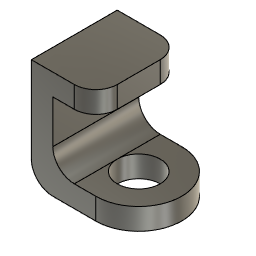
excercise 3 (Autodesk Fusion 360 design; units mm, degrees)
Autodesk Fusion 360 part; units mm, degrees
sketch "Sketch2" plane through (0, 0, 0) normal (0, 1, 0) x (1, 0, 0)
  line L0 (0, -10) -> (0, -50.06)
  line L1 (0, -50.06) -> (30, -50.06)
  line L2 (30, -50.06) -> (30, -40.06)
  line L3 (10, 0) -> (50, 0)
  line L4 (50, 0) -> (50, -10)
  arc A0 (10, 0) -> (0, -10) centre (10, -10) ccw
  line L5 (50, -10) -> (20, -10)
  line L6 (30, -40.06) -> (10, -40.06)
  line L7 (10, -40.06) -> (10, -20)
  arc A1 (20, -10) -> (10, -20) centre (20, -20) ccw
  point P0 (10, -10)
  dimension "d9" = 50.06
  dimension "d10" = 30
  dimension "d11" = 10
  dimension "d12" = 50
  dimension "d13" = 10
  dimension "d14" = 10
  dimension "d15" = 40
  dimension "d16" = 20
  dimension "d17" = 10
  constraint vertical L0
  constraint perpendicular L0 L1
  constraint perpendicular L1 L2
  constraint perpendicular L0 L3
  constraint perpendicular L3 L4
  constraint coincident origin L0
  constraint coincident origin L3
  constraint tangent L0 A0
  constraint tangent L3 A0
  constraint perpendicular L4 L5
  constraint perpendicular L2 L6
  constraint coincident P0 L5
  constraint tangent L7 A1
  constraint tangent L5 A1
  measures "d9" distance of origin L0.end
  measures "d10" distance of L0.end L1.end
  measures "d11" distance of L1.end L2.end
  measures "d12" distance of origin L3.end
  measures "d13" distance of L3.end L4.end
  measures "d14" radius of A0
  measures "d15" distance of L4.end P0
  measures "d16" distance of L2.end L6.end
  measures "d17" radius of A1
extrude "Extrude1" add sketch "Sketch2" along normal blind 40
sketch "Sketch5" plane through (0, 0, 50.06) normal (0, 0, 1) x (-1, 0, 0)
  line L0 (0, 0) -> (-30, 0)
  line L1 (-30, 0) -> (-30, -40)
  line L2 (-30, -40) -> (0, -40)
  line L3 (0, -40) -> (0, 0)
  line L4 (0, 0) -> (-20, 0)
  line L5 (-30, -10) -> (-30, -30)
  line L6 (-20, -40) -> (0, -40)
  line L7 (0, -40) -> (0, 0)
  arc A0 (-30, -30) -> (-20, -40) centre (-20, -30) ccw
  arc A1 (-20, 0) -> (-30, -10) centre (-20, -10) ccw
  dimension "d24" = 10
  dimension "d25" = 10
  constraint horizontal L4
  constraint vertical L5
  constraint horizontal L6
  constraint vertical L7
  constraint coincident L0.start L3.end
  constraint tangent L6 A0
  constraint tangent L5 A0
  constraint tangent L4 A1
  constraint tangent L5 A1
  measures "d24" radius of A0
  measures "d25" radius of A1
extrude "Extrude2" cut sketch "Sketch5" against normal blind 10 contours L0 L1 A1
extrude "Extrude3" cut sketch "Sketch5" against normal blind 10 contours L1 L2 A0
sketch "Sketch6" plane through (0, 0, 10) normal (0, 0, 1) x (-1, 0, 0)
  line L0 (-20, 0) -> (-50, 0)
  line L1 (-50, 0) -> (-50, -40)
  line L2 (-50, -40) -> (-20, -40)
  line L3 (-20, -40) -> (-20, 0)
  line L4 (-20, 0) -> (-30, 0)
  circle A0 centre (-30, -20) radius 10
  circle A1 centre (-30, -20) radius 20
  dimension "d30" = 10
  constraint coincident L0.start L3.end
  constraint perpendicular L3 L4
  constraint tangent L3 A0
  constraint concentric A0 A1
  constraint tangent L1 A1
  measures "d30" distance of L0.start L4.end
extrude "Extrude4" cut sketch "Sketch6" against normal blind 10 contours A0
extrude "Extrude5" cut sketch "Sketch6" against normal blind 10 contours L0 L1 A1
extrude "Extrude6" cut sketch "Sketch6" against normal blind 10 contours L1 L2 A1
